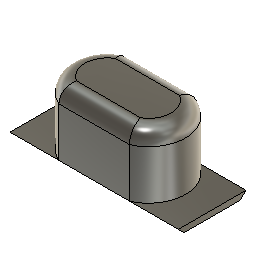
button (Autodesk Fusion 360 design; units mm, degrees)
Autodesk Fusion 360 part; units mm, degrees
sketch "Sketch1" plane through (0, 0, 0) normal (0, 0, 1) x (1, 0, 0)
  arc A0 (2.4187, -2.2) -> (2.4187, 2.2) centre (1.4436, 0) ccw
  line L0 (-2.4187, 2.2) -> (2.4187, 2.2)
  arc A1 (-2.4187, 2.2) -> (-2.4187, -2.2) centre (-1.4436, 0) ccw
  line L1 (2.4187, -2.2) -> (-2.4187, -2.2)
  line L2 (6.85, -2.55) -> (-6.85, -2.55)
  line L3 (-6.85, 2.55) -> (-6.85, -2.55)
  line L4 (6.85, 2.55) -> (-6.85, 2.55)
  line L5 (6.85, 2.55) -> (6.85, -2.55)
  arc A2 (2.45, -2.35) -> (2.45, 2.35) centre (1.4436, 0) ccw
  line L6 (-2.45, 2.35) -> (2.45, 2.35)
  arc A3 (-2.45, 2.35) -> (-2.45, -2.35) centre (-1.4436, 0) ccw
  line L7 (2.45, -2.35) -> (-2.45, -2.35)
  dimension "d33" = 0.15
extrude "Extrude3" add sketch "Sketch1" against normal blind 0.4 contours A0 L0 A1 L1 | L2 L3 L4 L5 | A2 L6 A3 L7
extrude "Extrude4" add sketch "Sketch1" along normal blind 4.4 contours A0 L0 A1 L1 | A2 L6 A3 L7
extrude "Extrude7" cut 1 faces at (6.85, 0.85, -0.1333) along direction (-1, 0, 0) blind 1
extrude "Extrude8" cut 1 faces at (-6.85, 0.85, -0.1333) along direction (1, 0, 0) blind 1
fillet "Fillet3" radius 1 4 edges at (-4, 0, 4.4) (0, -2.35, 4.4) (0, 2.35, 4.4) (4, 0, 4.4)
extrude "Extrude9" cut 1 faces at (-1.95, -2.55, -0.2667) along direction (0, 1, 0) up to surface (0.2 mm away)
extrude "Extrude10" cut 1 faces at (-1.95, 2.55, -0.2667) along direction (0, -1, 0) up to surface (0.2 mm away)
sketch "Sketch2" plane through (0, -2.35, 0) normal (0, -1, 0) x (1, 0, 0)
  line L0 (2.45, 3.4) -> (-2.45, 3.4)
  line L1 (-2.45, 3.4) -> (-2.45, 0)
  line L2 (-2.45, 0) -> (-5.85, 0)
  line L3 (-5.85, 0) -> (-5.85, -0.4)
  line L4 (-5.85, -0.4) -> (5.85, -0.4)
  line L5 (5.85, -0.4) -> (5.85, 0)
  line L6 (5.85, 0) -> (2.45, 0)
  line L7 (2.45, 0) -> (2.45, 3.4)
  line L8 (-2.45, 0) -> (2.45, 0)
  constraint coincident L1.end L2.start
  constraint coincident L6.end L7.start
sketch "Sketch3" plane through (0, 2.35, 0) normal (0, 1, 0) x (-1, 0, 0)
  line L0 (2.45, 3.4) -> (-2.45, 3.4)
  line L1 (-2.45, 3.4) -> (-2.45, 0)
  line L2 (-2.45, 0) -> (-5.85, 0)
  line L3 (-5.85, 0) -> (-5.85, -0.4)
  line L4 (-5.85, -0.4) -> (5.85, -0.4)
  line L5 (5.85, -0.4) -> (5.85, 0)
  line L6 (5.85, 0) -> (2.45, 0)
  line L7 (2.45, 0) -> (2.45, 3.4)
  line L8 (-2.45, 0) -> (2.45, 0)
  constraint coincident L1.end L2.start
  constraint coincident L6.end L7.start
chamfer "Chamfer2" distance 0.4 angle 45 2 edges at (0, 2.35, -0.4) (0, -2.35, -0.4)
